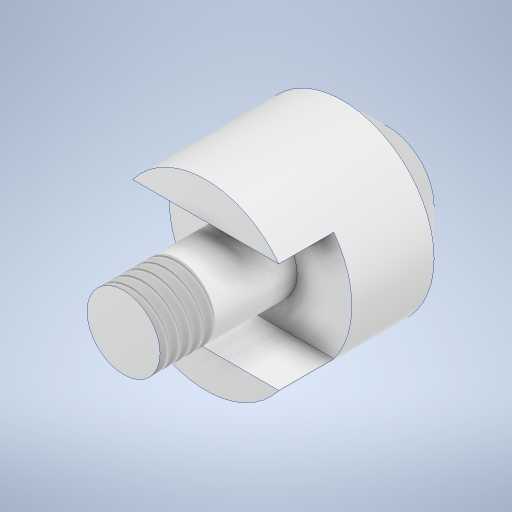
# Autodesk Inventor part: Część_1
Saved by Autodesk Inventor 2024 (Build 280153000, 153)
## iProperties
Created: 2024-04-13
Part Number: Część_1
Material: Aluminum 6061
Document SubType Name: Modeling
Designer: HP
Density: 2.7 g/cm^3
Appearance: Aluminum - Flat
Author: HP
Autodesk Inventor part; units mm, degrees
ref_plane "YZ Plane" through (0, 0, 0) normal (1, 0, 0) x (0, 1, 0)
ref_plane "XZ Plane" through (0, 0, 0) normal (0, 1, 0) x (-1, 0, 0)
ref_plane "XY Plane" through (0, 0, 0) normal (0, 0, 1) x (1, 0, 0)
sketch "Sketch1" plane through (0, 0, 0) normal (0, 0, 1) x (1, 0, 0)
  circle A0 centre (0, 0) radius 10
  dimension "d0" = 20
  constraints: 1 centre point, 1 coincident
  measures "d0" diameter of A0
extrude "Extrusion1" add sketch "Sketch1" along normal blind 18
sketch "Sketch2" plane through (0, 0, 18) normal (0, 0, 1) x (1, 0, 0)
  line L0 (0, 0) -> (0, 4) construction
  line L1 (0, 4) -> (-9.1652, 4)
  circle A0 centre (0, 0) radius 10 projected
  line L2 (0, 4) -> (9.1652, 4)
  line L3 (0, 0) -> (0, -4) construction
  line L4 (0, -4) -> (9.1652, -4)
  line L5 (0, -4) -> (-6.1702, -4)
  point P0 (-8, -6)
  dimension "d3" = 4
  dimension "d4" = 4
  constraints: 12 end point, 4 point on circle, 2 perpendicular, 2 point on line, 1 horizontal, 1 vertical
  measures "d3" distance of L0.start L0.end
  measures "d4" distance of L3.start L3.end
extrude "Extrusion2" cut sketch "Sketch2" against normal blind 4
sketch "Sketch3" plane through (0, 0, 0) normal (0, 0, -1) x (-1, 0, 0)
  circle A0 centre (0, 0) radius 3
  dimension "d7" = 6
  constraints: 1 centre point, 1 coincident
  measures "d7" diameter of A0
extrude "Extrusion3" cut sketch "Sketch3" against normal blind 10
thread "Thread1" size "M6x1" class "6H" standard "ANSI Metric M Profile" full length
sketch "Sketch7" plane through (0, 0, 14) normal (0, 0, 1) x (1, 0, 0)
  line L0 (0, 0) -> (0, -6) construction
  line L1 (0, -6) -> (-8, -6)
  circle A0 centre (0, 0) radius 10 projected
  line L2 (0, -6) -> (8, -6)
  line L3 (8, 6) -> (-8, 6)
  dimension "d21" = 6
  constraints: 8 end point, 4 point on circle, 1 parallel, 1 perpendicular, 1 point on line, 1 vertical
  measures "d21" distance of L0.start L0.end
extrude "Extrusion5" add sketch "Sketch7" along normal blind 6 contours L2 A0 L1 | A0 L3
sketch "Sketch8" plane through (0, 0, 14) normal (0, 0, 1) x (1, 0, 0)
  circle A0 centre (0, 0) radius 4
  dimension "d24" = 8
  constraints: 1 centre point, 1 coincident
  measures "d24" diameter of A0
extrude "Extrusion6" add sketch "Sketch8" along normal blind 15
thread "Thread4" size "M8x1.25" class "6g" standard "ANSI Metric M Profile" length 6
chamfer "Chamfer1" distance 5 angle 45 1 edges at (-10, 0, 0)
body "Solid1"
